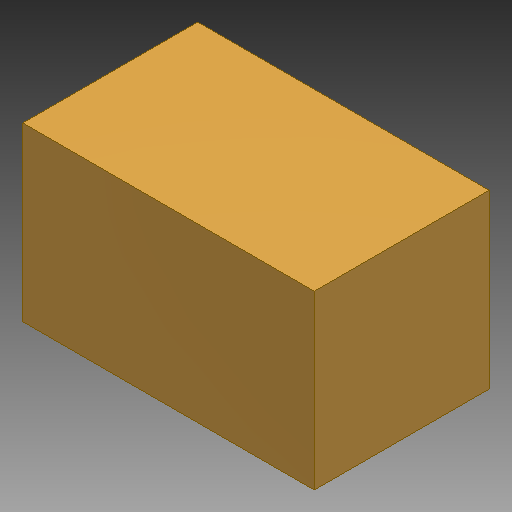
# Autodesk Inventor part: ML6
Saved by Autodesk Inventor 2017.3 (Build 213256000, 256)
## iProperties
Part Number: ML6
Material: Generisch
Document SubType Name: Modeling
Designer: Nils
Density: 1 g/cm^3
Appearance: ML6, ML6
Author: Nils
Autodesk Inventor part; units mm, degrees
ref_plane "YZ Plane" through (0, 0, 0) normal (1, 0, 0) x (0, 1, 0)
ref_plane "XZ Plane" through (0, 0, 0) normal (0, 1, 0) x (-1, 0, 0)
ref_plane "XY Plane" through (0, 0, 0) normal (0, 0, 1) x (1, 0, 0)
sketch "ML6, ML6_17" plane through (0, 0, 0) normal (0, 0, 1) x (1, 0, 0)
  line L0 (-7.62, 4.699) -> (7.62, 4.699)
  line L1 (7.62, 4.699) -> (7.62, -4.445)
  line L2 (7.62, -4.445) -> (-7.62, -4.445)
  line L3 (-7.62, -4.445) -> (-7.62, 4.699)
  constraints: 8 end point
extrude "Extrusion1" add sketch "ML6, ML6_17" along normal blind 9
